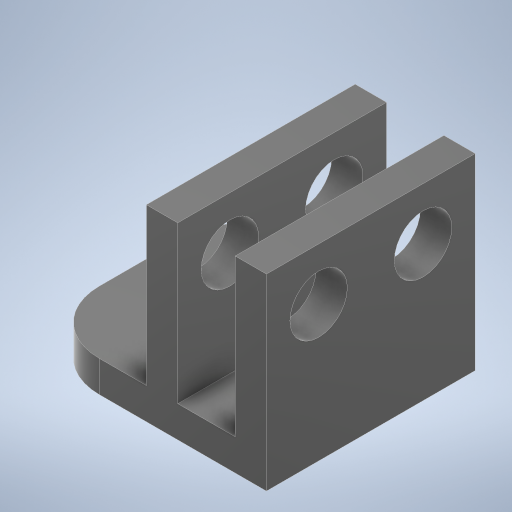
# Autodesk Inventor part: XY_Zfixer
Saved by Autodesk Inventor 2023 (Build 270158000, 158)
## iProperties
Created: 2023-11-27
Part Number: XY_Zfixer
Material: Thermoplastic Resin
Document SubType Name: Modeling
Designer: Mustapha
Density: 1.28 g/cm^3
Appearance: Smooth - Black
Mass: 3.43588 g
Surface Area: 24.9667 cm^2
Volume: 2.68428 cm^3
Author: Mustapha
Autodesk Inventor part; units mm, degrees
ref_plane "YZ Plane" through (0, 0, 0) normal (1, 0, 0) x (0, 1, 0)
ref_plane "XZ Plane" through (0, 0, 0) normal (0, 1, 0) x (-1, 0, 0)
ref_plane "XY Plane" through (0, 0, 0) normal (0, 0, 1) x (1, 0, 0)
sketch "Sketch1" plane through (0, 0, 0) normal (0, 1, 0) x (-1, 0, 0)
  line L0 (0, 0) -> (22, 0)
  line L1 (22, 0) -> (22, -20)
  line L2 (22, -20) -> (0, -20)
  line L3 (0, -20) -> (0, 0)
  dimension "d2" = 20
  dimension "d3" = 22
  constraints: 8 end point, 2 parallel, 1 horizontal, 1 perpendicular
  measures "d2" distance between parallel lines of L2 L0
  measures "d3" distance between parallel lines of L3 L1
extrude "Extrusion1" add sketch "Sketch1" along normal blind 3
sketch "Sketch3" plane through (0, 3, 0) normal (0, 1, 0) x (1, 0, 0)
  line L0 (0, 0) -> (-3, 0)
  line L1 (-3, 0) -> (-3, 20)
  line L2 (-3, 20) -> (0, 20)
  line L3 (0, 20) -> (0, 0)
  line L4 (-22, 0) -> (0, 0) projected
  line L5 (0, 20) -> (-22, 20) projected
  line L6 (-11.5, 0) -> (-8.5, 0)
  line L7 (-8.5, 0) -> (-8.5, 20)
  line L8 (-8.5, 20) -> (-11.5, 20)
  line L9 (-11.5, 20) -> (-11.5, 0)
  dimension "d8" = 3
  dimension "d25" = 3
  dimension "d26" = 5.5
  constraints: 16 end point, 4 parallel, 2 horizontal, 2 perpendicular, 2 point on line
  measures "d8" distance between parallel lines of L3 L1
  measures "d25" distance between parallel lines of L7 L9
  measures "d26" distance between parallel lines of L7 L1
extrude "Extrusion2" add sketch "Sketch3" along normal blind 15 contours L0 L1 L2 L3 | L4 L9 L5 L7
sketch "Sketch4" plane through (0, 0, 0) normal (1, 0, 0) x (0, 0, -1)
  line L0 (0, 3) -> (0, 18) projected
  line L1 (0, 13) -> (20.043, 13)
  line L2 (0, 18) -> (20, 18) projected
  circle A0 centre (5, 13) radius 2.75
  circle A1 centre (15, 13) radius 2.75
  line L3 (20, 0) -> (20, 18) projected
  point P0 (0, 0)
  dimension "d11" = 5
  dimension "d12" = 10
  dimension "d13" = 5.5
  dimension "d14" = 5.5
  dimension "d15" = 5
  constraints: 3 point on line, 2 centre point, 2 end point, 1 horizontal
  measures "d11" distance between parallel lines of L1 L2
  measures "d12" vertical distance of A0.centre L0
  measures "d13" diameter of A1
  measures "d14" diameter of A0
  measures "d15" distance from line of L3 A1.centre
extrude "Extrusion3" cut sketch "Sketch4" against normal blind 29.25 contours A0 L1 | L1 A0 | A1 L1 | L1 A1
sketch "Sketch5" plane through (0, 0, 0) normal (0, -1, 0) x (1, 0, 0)
  line L0 (-22, 0) -> (0, 0) projected
  line L1 (-16, 0) -> (-16, -20)
  line L2 (0, -20) -> (-22, -20) projected
  line L3 (-22, -20) -> (-22, 0) projected
  circle A0 centre (-16, -10) radius 4.25
  dimension "d18" = 6
  dimension "d19" = 8.5
  dimension "d27" = 10
  constraints: 2 end point, 2 point on line, 1 centre point, 1 midpoint, 1 vertical
  measures "d18" distance between parallel lines of L3 L1
  measures "d19" diameter of A0
  measures "d27" distance from line of L0 A0.centre
extrude "Extrusion4" cut sketch "Sketch5" against normal blind 1 contours A0 L1 | L1 A0
sketch "Sketch6" plane through (-16, 1, -10) normal (0, -1, 0) x (1, 0, 0)
  circle A0 centre (0, 0) radius 2.75
  point P0 (16, 10)
  dimension "d22" = 5.5
  constraints: 1 centre point
  measures "d22" diameter of A0
extrude "Extrusion5" cut sketch "Sketch6" against normal blind 9
fillet "Fillet1" radius 6 2 edges at (-22, 1.5, -20) (-22, 1.5, 0)
body "Solid1"
